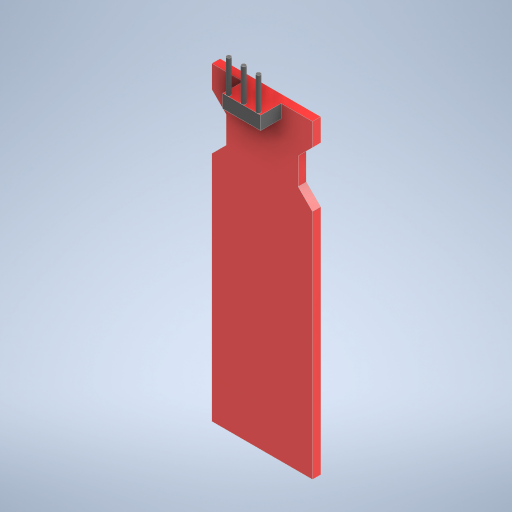
# Autodesk Inventor part: Water Sensor
Saved by Autodesk Inventor 2023 (Build 270158000, 158)
## iProperties
Created: 2023-09-26
Part Number: Water Sensor
Material: Generic
Document SubType Name: Modeling
Designer: Gage
Density: 1 g/cm^3
Appearance: Gray
Author: Gage
Autodesk Inventor part; units mm, degrees
ref_plane "YZ Plane" through (0, 0, 0) normal (1, 0, 0) x (0, 1, 0)
ref_plane "XZ Plane" through (0, 0, 0) normal (0, 1, 0) x (-1, 0, 0)
ref_plane "XY Plane" through (0, 0, 0) normal (0, 0, 1) x (1, 0, 0)
sketch "Sketch1" plane through (0, 0, 0) normal (0, 0, 1) x (1, 0, 0)
  line L0 (-9.7234, 29.9641) -> (9.7234, 29.9641)
  line L1 (9.7234, 29.9641) -> (9.7234, -29.9641)
  line L2 (9.7234, -29.9641) -> (-9.7234, -29.9641)
  line L3 (-9.7234, -29.9641) -> (-9.7234, 29.9641)
  point P0 (0, 0)
  point P1 (9.7234, 0)
  point P2 (0, -29.9641)
  dimension "d0" = 19.4469
  dimension "d1" = 59.9281
  constraints: 8 end point, 2 midpoint, 2 parallel, 1 horizontal, 1 horizontal alignment, 1 perpendicular, 1 vertical alignment
  measures "d0" distance of L1.end L2.end
  measures "d1" distance of L0.end L1.end
extrude "Extrusion1" add sketch "Sketch1" along normal blind 1.5875
sketch "Sketch2" plane through (0, 0, 1.5875) normal (0, 0, 1) x (1, 0, 0)
  line L0 (-9.7234, -29.9641) -> (9.7234, -29.9641) projected
  line L1 (9.7234, -29.9641) -> (9.7234, 14.8828)
  line L2 (9.7234, -29.9641) -> (9.7234, 29.9641) projected
  line L3 (-9.7234, 29.9641) -> (-9.7234, -29.9641) projected
  line L4 (-9.7234, -29.9641) -> (-9.7234, 14.8828)
  line L5 (-9.7234, 14.8828) -> (-0.7937, 23.8125)
  line L6 (-9.7234, 14.8828) -> (2.905, 14.8828) construction
  line L7 (9.7234, 14.8828) -> (4.7625, 19.8437)
  line L8 (9.7234, 14.8828) -> (16.7393, 14.8828) construction
  line L9 (6.9453, 22.8203) -> (6.9453, 17.6609)
  line L10 (-6.9453, 22.8203) -> (-6.9453, 17.6609)
  line L11 (-6.9453, 22.8203) -> (-9.7234, 25.5984)
  line L12 (6.9453, 22.8203) -> (9.7234, 25.5984)
  line L13 (-9.7234, 25.5984) -> (-9.7234, 14.8828)
  line L14 (9.7234, 25.5984) -> (9.7234, 14.8828)
  point P0 (0, 0)
  dimension "d4" = 44.8469
  dimension "d5" = 44.8469
  dimension "d6" = 45
  dimension "d7" = 135
  dimension "d8" = 5.1594
  dimension "d9" = 5.1594
  dimension "d10" = 2.7781
  dimension "d11" = 2.7781
  dimension "d12" = 0
  dimension "d13" = 0
  constraints: 24 end point, 5 point on line, 2 equal length, 2 horizontal, 2 vertical
  measures "d4" distance of L0.end L1.end
  measures "d5" distance of L0.start L4.end
  measures "d6" angle of L6 L5
  measures "d7" angle of L8 L7
  measures "d8" distance of L9.start L9.end
  measures "d9" distance of L10.start L10.end
  measures "d10" distance between parallel lines of L2 L9
  measures "d11" distance between parallel lines of L3 L10
  measures "d12" distance from line of L7 L9.end
  measures "d13" distance from line of L5 L10.end
extrude "Extrusion2" cut sketch "Sketch2" against normal blind 1.5875
sketch "Sketch3" plane through (0, 0, 1.5875) normal (0, 0, 1) x (1, 0, 0)
  line L0 (9.7234, 29.9641) -> (-9.7234, 29.9641) projected
  line L1 (-3.6711, 29.9641) -> (3.6711, 29.9641)
  line L2 (3.6711, 29.9641) -> (3.6711, 27.3844)
  line L3 (3.6711, 27.3844) -> (-3.6711, 27.3844)
  line L4 (-3.6711, 27.3844) -> (-3.6711, 29.9641)
  point P0 (0, 0)
  point P1 (0, 27.3844)
  dimension "d16" = 7.3422
  dimension "d17" = 2.5797
  constraints: 8 end point, 2 parallel, 1 horizontal, 1 midpoint, 1 perpendicular, 1 point on line, 1 vertical alignment
  measures "d16" distance of L2.end L3.end
  measures "d17" distance of L1.end L2.end
extrude "Extrusion3" add sketch "Sketch3" along normal blind 3.9688
sketch "Sketch4" plane through (-9.7234, 29.9641, 0) normal (0, 1, 0) x (1, 0, 0)
  circle A0 centre (12.6008, -5.1594) radius 0.3969
  circle A1 centre (9.7226, -5.1594) radius 0.3969
  circle A2 centre (6.8461, -5.1594) radius 0.3969
  line L0 (13.3945, -1.5875) -> (13.3945, -5.5563) projected
  line L1 (13.3945, -5.5563) -> (6.0523, -5.5563) projected
  line L2 (6.0523, -1.5875) -> (6.0523, -5.5563) projected
  point P0 (9.7234, 0)
  dimension "d20" = 0.7937
  dimension "d21" = 0.7937
  dimension "d22" = 0.7937
  dimension "d23" = 0.7937
  dimension "d24" = 0.3969
  dimension "d25" = 0.7937
  dimension "d26" = 0.3969
  dimension "d27" = 0.3969
  dimension "d28" = 7.3422
  dimension "d29" = 3.6703
  constraints: 3 centre point
  measures "d20" diameter of A0
  measures "d21" diameter of A1
  measures "d22" diameter of A2
  measures "d23" distance from line of L0 A0.centre
  measures "d24" distance from line of L1 A0.centre
  measures "d25" distance from line of L2 A2.centre
  measures "d26" distance from line of L1 A2.centre
  measures "d27" distance from line of L1 A1.centre
  measures "d28" distance between parallel lines of L2 L0
  measures "d29" distance from line of L2 A1.centre
extrude "Extrusion4" add sketch "Sketch4" along normal blind 6.35
body "Solid1"
